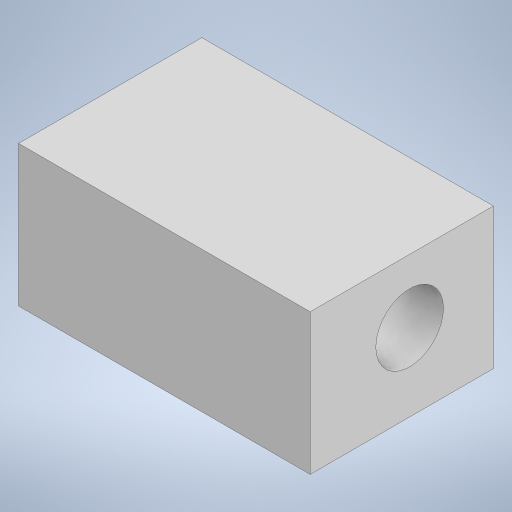
# Autodesk Inventor part: Pieza para tornillos
Saved by Autodesk Inventor 2024 (Build 280153000, 153)
## iProperties
Created: 2026-01-08
Part Number: Pieza para tornillos
Material: Generic
Document SubType Name: Modeling
Designer: eduso
Density: 1 g/cm^3
Appearance: Default
Author: eduso
Autodesk Inventor part; units mm, degrees
ref_plane "YZ Plane" through (0, 0, 0) normal (1, 0, 0) x (0, 1, 0)
ref_plane "XZ Plane" through (0, 0, 0) normal (0, 1, 0) x (-1, 0, 0)
ref_plane "XY Plane" through (0, 0, 0) normal (0, 0, 1) x (1, 0, 0)
sketch "Sketch1" plane through (0, 0, 0) normal (1, 0, 0) x (0, 1, 0)
  line L0 (-14.5623, 18.9434) -> (14.5623, 18.9434)
  line L1 (14.5623, 18.9434) -> (14.5623, -18.9434)
  line L2 (14.5623, -18.9434) -> (-14.5623, -18.9434)
  line L3 (-14.5623, -18.9434) -> (-14.5623, 18.9434)
  line L4 (-14.5623, 18.9434) -> (14.5623, -18.9434) construction
  line L5 (14.5623, 18.9434) -> (-14.5623, -18.9434) construction
  point P0 (0, 0)
  constraints: 12 end point, 2 midpoint, 2 parallel, 1 horizontal, 1 perpendicular
extrude "Extrusion1" add sketch "Sketch1" along normal blind 60.3
sketch "Sketch2" plane through (60.3, 0, 0) normal (1, 0, 0) x (0, 0, -1)
  point P0 (0, 0)
  point P1 (1.6165, 1.4208)
hole "Hole1" at (60.3, 1.4208, -1.6165) direction (-1, 0, 0) diameter 14 end through all
body "Solid1"
